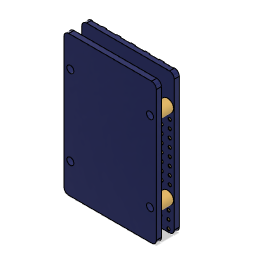
F405wse (Autodesk Fusion 360 design; units mm, degrees)
Autodesk Fusion 360 part; units mm, degrees
note: some values were not read from the file. Set by a fixed rule: which sketch regions a step uses.
sketch "Skizze1" plane through (0, 0, 0) normal (0, 0, 1) x (1, 0, 0)
  line L0 (-14.5, 22) -> (14.5, 22)
  line L1 (14.5, 22) -> (14.5, -22)
  line L2 (14.5, -22) -> (-14.5, -22)
  line L3 (-14.5, -22) -> (-14.5, 22)
  line L4 (-14.5, 22) -> (14.5, -22) construction
  line L5 (14.5, 22) -> (-14.5, -22) construction
  line L6 (-12.5, 12.5) -> (12.5, 12.5) construction
  line L7 (12.5, 12.5) -> (12.5, -12.5) construction
  line L8 (12.5, -12.5) -> (-12.5, -12.5) construction
  line L9 (-12.5, -12.5) -> (-12.5, 12.5) construction
  line L10 (-12.5, 12.5) -> (12.5, -12.5) construction
  line L11 (12.5, 12.5) -> (-12.5, -12.5) construction
  circle A0 centre (-12.5, 12.5) radius 1.1
  circle A1 centre (12.5, 12.5) radius 1.1
  circle A2 centre (12.5, -12.5) radius 1.1
  circle A3 centre (-12.5, -12.5) radius 1.1
  dimension "d1" = 29
  dimension "d2" = 44
  dimension "d7" = 25
  dimension "d8" = 25
  dimension "d9" = 2.2
  constraint horizontal L0
  constraint perpendicular L0 L1
  constraint parallel L0 L2
  constraint parallel L1 L3
  constraint coincident L4 origin
  constraint coincident L5 origin
  constraint horizontal L6
  constraint perpendicular L6 L7
  constraint parallel L6 L8
  constraint parallel L7 L9
  constraint coincident L10 origin
  constraint coincident L11 origin
  constraint coincident L6.start L9.end
  constraint coincident L6.end L7.start
  constraint coincident L7.end L8.start
  constraint coincident L8.end L9.start
  constraint equal A0 A1
  constraint equal A1 A2
  constraint equal A0 A3
  measures "d1" distance of L1.end L2.end
  measures "d2" distance of L0.end L1.end
  measures "d7" distance of L7.end L8.end
  measures "d8" distance of L6.end L7.end
  measures "d9" diameter of A0
extrude "Extrusion1" add sketch "Skizze1" along normal blind 1.2 makes body 1
fillet "Abrundung1" radius 1.5 4 edges at (-14.5, -22, 0.6) (14.5, -22, 0.6) (14.5, 22, 0.6) (-14.5, 22, 0.6) on bodies 1
sketch "Skizze3" plane through (0, 0, 0) normal (0, 0, -1) x (-1, 0, 0)
  arc A0 (14.5, 20.5) -> (13, 22) centre (13, 20.5) ccw
  line L0 (13, 22) -> (-13, 22)
  arc A1 (-13, 22) -> (-14.5, 20.5) centre (-13, 20.5) ccw
  line L1 (-14.5, 20.5) -> (-14.5, -20.5)
  arc A2 (-14.5, -20.5) -> (-13, -22) centre (-13, -20.5) ccw
  line L2 (-13, -22) -> (13, -22)
  arc A3 (13, -22) -> (14.5, -20.5) centre (13, -20.5) ccw
  line L3 (14.5, -20.5) -> (14.5, 20.5)
  circle A4 centre (-12.5, -12.5) radius 1.1
  circle A5 centre (12.5, -12.5) radius 1.1
  circle A6 centre (-12.5, 12.5) radius 1.1
  circle A7 centre (12.5, 12.5) radius 1.1
  line L4 (-0.75, 22) -> (-3.75, 22)
  line L5 (-3.75, 22) -> (-3.75, 19)
  line L6 (-3.75, 19) -> (-0.75, 19)
  line L7 (-0.75, 19) -> (-0.75, 22)
  line L8 (-12.75, 22) -> (-12.75, 19)
  line L9 (-12.75, 19) -> (-9.75, 19)
  line L10 (-9.75, 22) -> (-12.75, 22)
  line L11 (-9.75, 19) -> (-9.75, 22)
  line L12 (-8.25, 22) -> (-8.25, 19)
  line L13 (-8.25, 19) -> (-5.25, 19)
  line L14 (-5.25, 22) -> (-8.25, 22)
  line L15 (-5.25, 19) -> (-5.25, 22)
  line L16 (0.75, 22) -> (0.75, 19)
  line L17 (0.75, 19) -> (3.75, 19)
  line L18 (3.75, 22) -> (0.75, 22)
  line L19 (3.75, 19) -> (3.75, 22)
  line L20 (5.25, 22) -> (5.25, 19)
  line L21 (5.25, 19) -> (8.25, 19)
  line L22 (8.25, 22) -> (5.25, 22)
  line L23 (8.25, 19) -> (8.25, 22)
  line L24 (9.75, 22) -> (9.75, 19)
  line L25 (9.75, 19) -> (12.75, 19)
  line L26 (12.75, 22) -> (9.75, 22)
  line L27 (12.75, 19) -> (12.75, 22)
  circle A8 centre (-8, -1.27) radius 0.5
  circle A9 centre (-8, -8.89) radius 0.5
  circle A10 centre (-10.54, -8.89) radius 0.5
  circle A11 centre (-13.08, -8.89) radius 0.5
  circle A12 centre (-8, -6.35) radius 0.5
  circle A13 centre (-10.54, -6.35) radius 0.5
  circle A14 centre (-13.08, -6.35) radius 0.5
  circle A15 centre (-8, -3.81) radius 0.5
  circle A16 centre (-10.54, -3.81) radius 0.5
  circle A17 centre (-13.08, -3.81) radius 0.5
  circle A18 centre (-10.54, -1.27) radius 0.5
  circle A19 centre (-13.08, -1.27) radius 0.5
  circle A20 centre (-8, 1.27) radius 0.5
  circle A21 centre (-10.54, 1.27) radius 0.5
  circle A22 centre (-13.08, 1.27) radius 0.5
  circle A23 centre (-8, 3.81) radius 0.5
  circle A24 centre (-10.54, 3.81) radius 0.5
  circle A25 centre (-13.08, 3.81) radius 0.5
  circle A26 centre (-8, 6.35) radius 0.5
  circle A27 centre (-10.54, 6.35) radius 0.5
  circle A28 centre (-13.08, 6.35) radius 0.5
  circle A29 centre (-8, 8.89) radius 0.5
  circle A30 centre (-10.54, 8.89) radius 0.5
  circle A31 centre (-13.08, 8.89) radius 0.5
  circle A32 centre (0, -16) radius 0.5
  circle A33 centre (-12.7, -16) radius 0.5
  circle A34 centre (-10.16, -16) radius 0.5
  circle A35 centre (-7.62, -16) radius 0.5
  circle A36 centre (-5.08, -16) radius 0.5
  circle A37 centre (-2.54, -16) radius 0.5
  circle A38 centre (2.54, -16) radius 0.5
  circle A39 centre (5.08, -16) radius 0.5
  circle A40 centre (7.62, -16) radius 0.5
  circle A41 centre (10.16, -16) radius 0.5
  circle A42 centre (12.7, -16) radius 0.5
  circle A43 centre (-12.7, -18.54) radius 0.5
  circle A44 centre (-10.16, -18.54) radius 0.5
  circle A45 centre (-7.62, -18.54) radius 0.5
  circle A46 centre (-5.08, -18.54) radius 0.5
  circle A47 centre (-2.54, -18.54) radius 0.5
  circle A48 centre (0, -18.54) radius 0.5
  circle A49 centre (2.54, -18.54) radius 0.5
  circle A50 centre (5.08, -18.54) radius 0.5
  circle A51 centre (7.62, -18.54) radius 0.5
  circle A52 centre (10.16, -18.54) radius 0.5
  circle A53 centre (12.7, -18.54) radius 0.5
  circle A54 centre (-12.7, -21.08) radius 0.5
  circle A55 centre (-10.16, -21.08) radius 0.5
  circle A56 centre (-7.62, -21.08) radius 0.5
  circle A57 centre (-5.08, -21.08) radius 0.5
  circle A58 centre (-2.54, -21.08) radius 0.5
  circle A59 centre (0, -21.08) radius 0.5
  circle A60 centre (2.54, -21.08) radius 0.5
  circle A61 centre (5.08, -21.08) radius 0.5
  circle A62 centre (7.62, -21.08) radius 0.5
  circle A63 centre (10.16, -21.08) radius 0.5
  circle A64 centre (12.7, -21.08) radius 0.5
  dimension "d33" = 3
  dimension "d34" = 3
  dimension "d35" = 0.75
  dimension "d38" = 4.5
  dimension "d39" = 0
  dimension "d40" = 1
  dimension "d43" = -2.54
  dimension "d44" = 2.54
  dimension "d45" = 1.27
  dimension "d46" = 8
  dimension "d49" = 2.54
  dimension "d50" = -2.54
  dimension "d51" = 16
  constraint horizontal L4
  constraint vertical L5
  constraint horizontal L6
  constraint vertical L7
  constraint coincident L0 L4.start
  constraint equal A8 A32
  constraint vertical origin A32.centre
  measures "d33" distance of L4.start L4.end
  measures "d34" distance of L4.start L6.end
  measures "d35" distance of origin L7
  measures "d40" diameter of A8
  measures "d45" vertical distance of origin A8.centre
  measures "d46" horizontal distance of origin A8.centre
  measures "d51" distance of origin A32.centre
extrude "Extrusion3" add sketch "Skizze3" along normal blind 0.2 contours A0 L0 A1 L1 A2 L2 A3 L3 L5 L6 L7 L8 L9 L11 L12 L13 L15 L16 L17 L19 L20 L21 L23 L24 L25 L27 bodies 1
sketch "Skizze4" plane through (0, 0, 1.2) normal (0, 0, 1) x (1, 0, 0)
  circle A0 centre (-12.5, -12.5) radius 1.1
  circle A1 centre (12.5, -12.5) radius 1.1
  circle A2 centre (12.5, 12.5) radius 1.1
  circle A3 centre (-12.5, 12.5) radius 1.1
  arc A4 (-13, 22) -> (-14.5, 20.5) centre (-13, 20.5) ccw
  line L0 (-14.5, 20.5) -> (-14.5, -20.5)
  arc A5 (-14.5, -20.5) -> (-13, -22) centre (-13, -20.5) ccw
  line L1 (-13, -22) -> (13, -22)
  arc A6 (13, -22) -> (14.5, -20.5) centre (13, -20.5) ccw
  line L2 (14.5, -20.5) -> (14.5, 20.5)
  arc A7 (14.5, 20.5) -> (13, 22) centre (13, 20.5) ccw
  line L3 (13, 22) -> (-13, 22)
  circle A8 centre (12.5, -12.5) radius 1.1
  circle A9 centre (12.5, 12.5) radius 1.1
  circle A10 centre (13.08, -6.35) radius 0.5
  circle A11 centre (10.54, -6.35) radius 0.5
  circle A12 centre (8, -6.35) radius 0.5
  circle A13 centre (8, -1.27) radius 0.5
  circle A14 centre (-12.5, 12.5) radius 1.1
  circle A15 centre (13.08, -8.89) radius 0.5
  circle A16 centre (8, -8.89) radius 0.5
  circle A17 centre (10.54, -8.89) radius 0.5
  circle A18 centre (8, -3.81) radius 0.5
  circle A19 centre (13.08, -3.81) radius 0.5
  circle A20 centre (10.54, -3.81) radius 0.5
  circle A21 centre (-12.5, -12.5) radius 1.1
  circle A22 centre (2.54, -21.08) radius 0.5
  circle A23 centre (12.7, -18.54) radius 0.5
  circle A24 centre (13.08, 8.89) radius 0.5
  circle A25 centre (13.08, 6.35) radius 0.5
  circle A26 centre (5.08, -16) radius 0.5
  circle A27 centre (-5.08, -16) radius 0.5
  circle A28 centre (-7.62, -21.08) radius 0.5
  circle A29 centre (7.62, -21.08) radius 0.5
  circle A30 centre (-12.7, -21.08) radius 0.5
  circle A31 centre (-10.16, -16) radius 0.5
  circle A32 centre (0, -16) radius 0.5
  circle A33 centre (13.08, 3.81) radius 0.5
  circle A34 centre (10.54, 1.27) radius 0.5
  circle A35 centre (13.08, 1.27) radius 0.5
  circle A36 centre (8, 6.35) radius 0.5
  circle A37 centre (7.62, -16) radius 0.5
  circle A38 centre (-5.08, -21.08) radius 0.5
  circle A39 centre (-2.54, -16) radius 0.5
  circle A40 centre (-7.62, -18.54) radius 0.5
  circle A41 centre (10.54, 8.89) radius 0.5
  circle A42 centre (10.54, 6.35) radius 0.5
  circle A43 centre (8, 3.81) radius 0.5
  circle A44 centre (8, 1.27) radius 0.5
  circle A45 centre (10.54, 3.81) radius 0.5
  circle A46 centre (8, 8.89) radius 0.5
  circle A47 centre (2.54, -16) radius 0.5
  circle A48 centre (-2.54, -21.08) radius 0.5
  circle A49 centre (-10.16, -18.54) radius 0.5
  circle A50 centre (12.7, -21.08) radius 0.5
  circle A51 centre (-12.7, -18.54) radius 0.5
  circle A52 centre (10.16, -21.08) radius 0.5
  circle A53 centre (5.08, -21.08) radius 0.5
  circle A54 centre (-10.16, -21.08) radius 0.5
  circle A55 centre (-7.62, -16) radius 0.5
  circle A56 centre (10.16, -16) radius 0.5
  circle A57 centre (10.54, -1.27) radius 0.5
  circle A58 centre (13.08, -1.27) radius 0.5
  circle A59 centre (12.7, -16) radius 0.5
  circle A60 centre (-12.7, -16) radius 0.5
  circle A61 centre (0, -21.08) radius 0.5
  circle A62 centre (-5.08, -18.54) radius 0.5
  circle A63 centre (7.62, -18.54) radius 0.5
  circle A64 centre (5.08, -18.54) radius 0.5
  circle A65 centre (-2.54, -18.54) radius 0.5
  circle A66 centre (2.54, -18.54) radius 0.5
  circle A67 centre (0, -18.54) radius 0.5
  circle A68 centre (10.16, -18.54) radius 0.5
  line L4 (-9.75, 22) -> (-8.25, 22)
  line L5 (-8.25, 22) -> (-8.25, 19)
  line L6 (-8.25, 19) -> (-5.25, 19)
  line L7 (-5.25, 19) -> (-5.25, 22)
  line L8 (-5.25, 22) -> (-3.75, 22)
  line L9 (-3.75, 22) -> (-3.75, 19)
  line L10 (-3.75, 19) -> (-0.75, 19)
  line L11 (-0.75, 19) -> (-0.75, 22)
  line L12 (-0.75, 22) -> (0.75, 22)
  line L13 (0.75, 22) -> (0.75, 19)
  line L14 (0.75, 19) -> (3.75, 19)
  line L15 (3.75, 19) -> (3.75, 22)
  line L16 (3.75, 22) -> (5.25, 22)
  line L17 (5.25, 22) -> (5.25, 19)
  line L18 (5.25, 19) -> (8.25, 19)
  line L19 (8.25, 19) -> (8.25, 22)
  line L20 (8.25, 22) -> (9.75, 22)
  line L21 (9.75, 22) -> (9.75, 19)
  line L22 (9.75, 19) -> (12.75, 19)
  line L23 (12.75, 19) -> (12.75, 22)
  line L24 (12.75, 22) -> (13, 22)
  arc A69 (14.5, 20.5) -> (13, 22) centre (13, 20.5) ccw
  line L25 (14.5, 20.5) -> (14.5, -20.5)
  arc A70 (13, -22) -> (14.5, -20.5) centre (13, -20.5) ccw
  line L26 (13, -22) -> (-13, -22)
  arc A71 (-14.5, -20.5) -> (-13, -22) centre (-13, -20.5) ccw
  line L27 (-14.5, -20.5) -> (-14.5, 20.5)
  arc A72 (-13, 22) -> (-14.5, 20.5) centre (-13, 20.5) ccw
  line L28 (-13, 22) -> (-12.75, 22)
  line L29 (-12.75, 22) -> (-12.75, 19)
  line L30 (-12.75, 19) -> (-9.75, 19)
  line L31 (-9.75, 19) -> (-9.75, 22)
extrude "Extrusion4" add sketch "Skizze4" along normal blind 0.2 bodies 1
sketch "Skizze5" plane through (0, 0, -0.2) normal (0, 0, -1) x (-1, 0, 0)
  circle A0 centre (-12.5, -12.5) radius 1.1
  circle A1 centre (-12.5, 12.5) radius 1.1
  circle A2 centre (-13.08, -6.35) radius 0.5
  circle A3 centre (-10.54, -6.35) radius 0.5
  circle A4 centre (-8, -6.35) radius 0.5
  circle A5 centre (-8, -1.27) radius 0.5
  circle A6 centre (12.5, 12.5) radius 1.1
  circle A7 centre (-13.08, -8.89) radius 0.5
  circle A8 centre (-8, -8.89) radius 0.5
  circle A9 centre (-10.54, -8.89) radius 0.5
  circle A10 centre (-8, -3.81) radius 0.5
  circle A11 centre (-13.08, -3.81) radius 0.5
  circle A12 centre (-10.54, -3.81) radius 0.5
  circle A13 centre (12.5, -12.5) radius 1.1
  circle A14 centre (-2.54, -21.08) radius 0.5
  circle A15 centre (-12.7, -18.54) radius 0.5
  circle A16 centre (-13.08, 8.89) radius 0.5
  circle A17 centre (-13.08, 6.35) radius 0.5
  circle A18 centre (-5.08, -16) radius 0.5
  circle A19 centre (5.08, -16) radius 0.5
  circle A20 centre (7.62, -21.08) radius 0.5
  circle A21 centre (-7.62, -21.08) radius 0.5
  circle A22 centre (12.7, -21.08) radius 0.5
  circle A23 centre (10.16, -16) radius 0.5
  circle A24 centre (0, -16) radius 0.5
  circle A25 centre (-13.08, 3.81) radius 0.5
  circle A26 centre (-10.54, 1.27) radius 0.5
  circle A27 centre (-13.08, 1.27) radius 0.5
  circle A28 centre (-8, 6.35) radius 0.5
  circle A29 centre (-7.62, -16) radius 0.5
  circle A30 centre (5.08, -21.08) radius 0.5
  circle A31 centre (2.54, -16) radius 0.5
  circle A32 centre (7.62, -18.54) radius 0.5
  circle A33 centre (-10.54, 8.89) radius 0.5
  circle A34 centre (-10.54, 6.35) radius 0.5
  circle A35 centre (-8, 3.81) radius 0.5
  circle A36 centre (-8, 1.27) radius 0.5
  circle A37 centre (-10.54, 3.81) radius 0.5
  circle A38 centre (-8, 8.89) radius 0.5
  circle A39 centre (-2.54, -16) radius 0.5
  circle A40 centre (2.54, -21.08) radius 0.5
  circle A41 centre (10.16, -18.54) radius 0.5
  circle A42 centre (-12.7, -21.08) radius 0.5
  circle A43 centre (12.7, -18.54) radius 0.5
  circle A44 centre (-10.16, -21.08) radius 0.5
  circle A45 centre (-5.08, -21.08) radius 0.5
  circle A46 centre (10.16, -21.08) radius 0.5
  circle A47 centre (7.62, -16) radius 0.5
  circle A48 centre (-10.16, -16) radius 0.5
  circle A49 centre (-10.54, -1.27) radius 0.5
  circle A50 centre (-13.08, -1.27) radius 0.5
  circle A51 centre (-12.7, -16) radius 0.5
  circle A52 centre (12.7, -16) radius 0.5
  circle A53 centre (0, -21.08) radius 0.5
  circle A54 centre (5.08, -18.54) radius 0.5
  circle A55 centre (-7.62, -18.54) radius 0.5
  circle A56 centre (-5.08, -18.54) radius 0.5
  circle A57 centre (2.54, -18.54) radius 0.5
  circle A58 centre (-2.54, -18.54) radius 0.5
  circle A59 centre (0, -18.54) radius 0.5
  circle A60 centre (-10.16, -18.54) radius 0.5
  line L0 (9.75, 22) -> (8.25, 22)
  line L1 (8.25, 22) -> (8.25, 19)
  line L2 (8.25, 19) -> (5.25, 19)
  line L3 (5.25, 19) -> (5.25, 22)
  line L4 (5.25, 22) -> (3.75, 22)
  line L5 (3.75, 22) -> (3.75, 19)
  line L6 (3.75, 19) -> (0.75, 19)
  line L7 (0.75, 19) -> (0.75, 22)
  line L8 (0.75, 22) -> (-0.75, 22)
  line L9 (-0.75, 22) -> (-0.75, 19)
  line L10 (-0.75, 19) -> (-3.75, 19)
  line L11 (-3.75, 19) -> (-3.75, 22)
  line L12 (-3.75, 22) -> (-5.25, 22)
  line L13 (-5.25, 22) -> (-5.25, 19)
  line L14 (-5.25, 19) -> (-8.25, 19)
  line L15 (-8.25, 19) -> (-8.25, 22)
  line L16 (-8.25, 22) -> (-9.75, 22)
  line L17 (-9.75, 22) -> (-9.75, 19)
  line L18 (-9.75, 19) -> (-12.75, 19)
  line L19 (-12.75, 19) -> (-12.75, 22)
  line L20 (-12.75, 22) -> (-13, 22)
  arc A61 (-13, 22) -> (-14.5, 20.5) centre (-13, 20.5) ccw
  line L21 (-14.5, 20.5) -> (-14.5, -20.5)
  arc A62 (-14.5, -20.5) -> (-13, -22) centre (-13, -20.5) ccw
  line L22 (-13, -22) -> (13, -22)
  arc A63 (13, -22) -> (14.5, -20.5) centre (13, -20.5) ccw
  line L23 (14.5, -20.5) -> (14.5, 20.5)
  arc A64 (14.5, 20.5) -> (13, 22) centre (13, 20.5) ccw
  line L24 (13, 22) -> (12.75, 22)
  line L25 (12.75, 22) -> (12.75, 19)
  line L26 (12.75, 19) -> (9.75, 19)
  line L27 (9.75, 19) -> (9.75, 22)
  line L28 (1, 6) -> (13, 6)
  line L29 (13, 6) -> (13, -6)
  line L30 (13, -6) -> (1, -6)
  line L31 (1, -6) -> (1, 6)
  dimension "d56" = 12
  dimension "d57" = 6
  dimension "d58" = 1
  constraint horizontal L28
  constraint vertical L29
  constraint horizontal L30
  constraint vertical L31
  constraint equal L28 L31
  measures "d56" distance of L28.start L28.end
  measures "d57" distance of origin L28
  measures "d58" distance of origin L31
extrude "Extrusion5" add sketch "Skizze5" along normal blind 2 contours L28 L29 L30 L31 bodies 1
chamfer "Fase1" distance 0.5 angle 45 4 edges at (-7, -6, -0.2) (-1, 0, -0.2) (-13, 0, -0.2) (-7, 6, -0.2) on bodies 1
sketch "Skizze6" plane through (0, 0, -0.2) normal (0, 0, -1) x (-1, 0, 0)
  line L0 (9.75, 22) -> (8.25, 22)
  line L1 (8.25, 22) -> (8.25, 19)
  line L2 (8.25, 19) -> (5.25, 19)
  line L3 (5.25, 19) -> (5.25, 22)
  line L4 (5.25, 22) -> (3.75, 22)
  line L5 (3.75, 22) -> (3.75, 19)
  line L6 (3.75, 19) -> (0.75, 19)
  line L7 (0.75, 19) -> (0.75, 22)
  line L8 (0.75, 22) -> (-0.75, 22)
  line L9 (-0.75, 22) -> (-0.75, 19)
  line L10 (-0.75, 19) -> (-3.75, 19)
  line L11 (-3.75, 19) -> (-3.75, 22)
  line L12 (-3.75, 22) -> (-5.25, 22)
  line L13 (-5.25, 22) -> (-5.25, 19)
  line L14 (-5.25, 19) -> (-8.25, 19)
  line L15 (-8.25, 19) -> (-8.25, 22)
  line L16 (-8.25, 22) -> (-9.75, 22)
  line L17 (-9.75, 22) -> (-9.75, 19)
  line L18 (-9.75, 19) -> (-12.75, 19)
  line L19 (-12.75, 19) -> (-12.75, 22)
  line L20 (-12.75, 22) -> (-13, 22)
  arc A0 (-13, 22) -> (-14.5, 20.5) centre (-13, 20.5) ccw
  line L21 (-14.5, 20.5) -> (-14.5, -20.5)
  arc A1 (-14.5, -20.5) -> (-13, -22) centre (-13, -20.5) ccw
  line L22 (-13, -22) -> (13, -22)
  arc A2 (13, -22) -> (14.5, -20.5) centre (13, -20.5) ccw
  line L23 (14.5, -20.5) -> (14.5, 20.5)
  arc A3 (14.5, 20.5) -> (13, 22) centre (13, 20.5) ccw
  line L24 (13, 22) -> (12.75, 22)
  line L25 (12.75, 22) -> (12.75, 19)
  line L26 (12.75, 19) -> (9.75, 19)
  line L27 (9.75, 19) -> (9.75, 22)
  circle A4 centre (-10.16, -18.54) radius 0.5
  circle A5 centre (0, -18.54) radius 0.5
  circle A6 centre (-2.54, -18.54) radius 0.5
  circle A7 centre (2.54, -18.54) radius 0.5
  circle A8 centre (-5.08, -18.54) radius 0.5
  circle A9 centre (-7.62, -18.54) radius 0.5
  circle A10 centre (5.08, -18.54) radius 0.5
  circle A11 centre (0, -21.08) radius 0.5
  circle A12 centre (12.7, -16) radius 0.5
  circle A13 centre (-12.7, -16) radius 0.5
  circle A14 centre (-13.08, -1.27) radius 0.5
  circle A15 centre (-10.54, -1.27) radius 0.5
  circle A16 centre (-10.16, -16) radius 0.5
  circle A17 centre (7.62, -16) radius 0.5
  circle A18 centre (10.16, -21.08) radius 0.5
  circle A19 centre (-5.08, -21.08) radius 0.5
  circle A20 centre (-10.16, -21.08) radius 0.5
  circle A21 centre (12.7, -18.54) radius 0.5
  circle A22 centre (-12.7, -21.08) radius 0.5
  circle A23 centre (10.16, -18.54) radius 0.5
  circle A24 centre (2.54, -21.08) radius 0.5
  circle A25 centre (-2.54, -16) radius 0.5
  circle A26 centre (-8, 8.89) radius 0.5
  circle A27 centre (-10.54, 3.81) radius 0.5
  circle A28 centre (-8, 1.27) radius 0.5
  circle A29 centre (-8, 3.81) radius 0.5
  circle A30 centre (-10.54, 6.35) radius 0.5
  circle A31 centre (-10.54, 8.89) radius 0.5
  circle A32 centre (7.62, -18.54) radius 0.5
  circle A33 centre (2.54, -16) radius 0.5
  circle A34 centre (5.08, -21.08) radius 0.5
  circle A35 centre (-7.62, -16) radius 0.5
  circle A36 centre (-8, 6.35) radius 0.5
  circle A37 centre (-13.08, 1.27) radius 0.5
  circle A38 centre (-10.54, 1.27) radius 0.5
  circle A39 centre (-13.08, 3.81) radius 0.5
  circle A40 centre (0, -16) radius 0.5
  circle A41 centre (10.16, -16) radius 0.5
  circle A42 centre (12.7, -21.08) radius 0.5
  circle A43 centre (-7.62, -21.08) radius 0.5
  circle A44 centre (7.62, -21.08) radius 0.5
  circle A45 centre (5.08, -16) radius 0.5
  circle A46 centre (-5.08, -16) radius 0.5
  circle A47 centre (-13.08, 6.35) radius 0.5
  circle A48 centre (-13.08, 8.89) radius 0.5
  circle A49 centre (-12.7, -18.54) radius 0.5
  circle A50 centre (-2.54, -21.08) radius 0.5
  circle A51 centre (12.5, -12.5) radius 1.1
  circle A52 centre (-10.54, -3.81) radius 0.5
  circle A53 centre (-13.08, -3.81) radius 0.5
  circle A54 centre (-8, -3.81) radius 0.5
  circle A55 centre (-10.54, -8.89) radius 0.5
  circle A56 centre (-8, -8.89) radius 0.5
  circle A57 centre (-13.08, -8.89) radius 0.5
  circle A58 centre (12.5, 12.5) radius 1.1
  circle A59 centre (-8, -1.27) radius 0.5
  circle A60 centre (-8, -6.35) radius 0.5
  circle A61 centre (-10.54, -6.35) radius 0.5
  circle A62 centre (-13.08, -6.35) radius 0.5
  circle A63 centre (-12.5, 12.5) radius 1.1
  circle A64 centre (-12.5, -12.5) radius 1.1
  line L28 (13.5, 6.5) -> (13.5, -6.5)
  line L29 (13.5, -6.5) -> (0.5, -6.5)
  line L30 (0.5, -6.5) -> (0.5, 6.5)
  line L31 (0.5, 6.5) -> (13.5, 6.5)
  line L32 (-6, 4) -> (-1, 4)
  line L33 (-1, 4) -> (-1, -8)
  line L34 (-1, -8) -> (-6, -8)
  line L35 (-6, -8) -> (-6, 4)
  dimension "d62" = 12
  dimension "d63" = 5
  dimension "d64" = 1
  dimension "d65" = 4
  constraint horizontal L32
  constraint vertical L33
  constraint horizontal L34
  constraint vertical L35
  measures "d62" distance of L32.start L34.end
  measures "d63" distance of L32.start L32.end
  measures "d64" distance of origin L33
  measures "d65" distance of origin L32
extrude "Extrusion6" add sketch "Skizze6" along normal blind 4 contours L32 L33 L34 L35 bodies 1
sketch "Skizze7" plane through (0, 0, 1.4) normal (0, 0, 1) x (1, 0, 0)
  circle A0 centre (-7.62, -21.08) radius 0.5
  circle A1 centre (12.5, -12.5) radius 1.1
  circle A2 centre (8, 8.89) radius 0.5
  circle A3 centre (8, 6.35) radius 0.5
  circle A4 centre (-10.16, -18.54) radius 0.5
  circle A5 centre (12.7, -21.08) radius 0.5
  circle A6 centre (10.16, -21.08) radius 0.5
  circle A7 centre (10.54, 3.81) radius 0.5
  circle A8 centre (7.62, -18.54) radius 0.5
  circle A9 centre (-12.5, 12.5) radius 1.1
  circle A10 centre (10.54, 1.27) radius 0.5
  circle A11 centre (-2.54, -16) radius 0.5
  circle A12 centre (10.54, 8.89) radius 0.5
  circle A13 centre (8, 3.81) radius 0.5
  circle A14 centre (5.08, -16) radius 0.5
  circle A15 centre (13.08, -6.35) radius 0.5
  circle A16 centre (12.7, -18.54) radius 0.5
  circle A17 centre (12.7, -16) radius 0.5
  circle A18 centre (-10.16, -16) radius 0.5
  circle A19 centre (0, -21.08) radius 0.5
  circle A20 centre (-12.7, -18.54) radius 0.5
  circle A21 centre (-2.54, -21.08) radius 0.5
  circle A22 centre (2.54, -16) radius 0.5
  circle A23 centre (8, -6.35) radius 0.5
  circle A24 centre (2.54, -21.08) radius 0.5
  circle A25 centre (-12.7, -21.08) radius 0.5
  circle A26 centre (13.08, 8.89) radius 0.5
  circle A27 centre (10.54, -6.35) radius 0.5
  circle A28 centre (8, -1.27) radius 0.5
  circle A29 centre (5.08, -18.54) radius 0.5
  circle A30 centre (8, -3.81) radius 0.5
  circle A31 centre (8, -8.89) radius 0.5
  circle A32 centre (13.08, 1.27) radius 0.5
  circle A33 centre (13.08, -8.89) radius 0.5
  circle A34 centre (0, -16) radius 0.5
  circle A35 centre (-5.08, -16) radius 0.5
  circle A36 centre (13.08, -3.81) radius 0.5
  circle A37 centre (-12.7, -16) radius 0.5
  circle A38 centre (7.62, -16) radius 0.5
  circle A39 centre (7.62, -21.08) radius 0.5
  circle A40 centre (-12.5, -12.5) radius 1.1
  circle A41 centre (13.08, -1.27) radius 0.5
  circle A42 centre (-5.08, -18.54) radius 0.5
  circle A43 centre (10.54, -3.81) radius 0.5
  circle A44 centre (10.16, -18.54) radius 0.5
  circle A45 centre (10.54, -8.89) radius 0.5
  circle A46 centre (13.08, 6.35) radius 0.5
  circle A47 centre (13.08, 3.81) radius 0.5
  circle A48 centre (-5.08, -21.08) radius 0.5
  circle A49 centre (-7.62, -18.54) radius 0.5
  circle A50 centre (10.54, 6.35) radius 0.5
  circle A51 centre (8, 1.27) radius 0.5
  circle A52 centre (-2.54, -18.54) radius 0.5
  circle A53 centre (10.54, -1.27) radius 0.5
  circle A54 centre (5.08, -21.08) radius 0.5
  circle A55 centre (2.54, -18.54) radius 0.5
  circle A56 centre (-10.16, -21.08) radius 0.5
  circle A57 centre (10.16, -16) radius 0.5
  circle A58 centre (-7.62, -16) radius 0.5
  circle A59 centre (0, -18.54) radius 0.5
  circle A60 centre (12.5, 12.5) radius 1.1
  arc A61 (-14.5, -20.5) -> (-13, -22) centre (-13, -20.5) ccw
  line L0 (-13, -22) -> (13, -22)
  arc A62 (13, -22) -> (14.5, -20.5) centre (13, -20.5) ccw
  line L1 (14.5, -20.5) -> (14.5, 20.5)
  arc A63 (14.5, 20.5) -> (13, 22) centre (13, 20.5) ccw
  line L2 (13, 22) -> (-13, 22)
  arc A64 (-13, 22) -> (-14.5, 20.5) centre (-13, 20.5) ccw
  line L3 (-14.5, 20.5) -> (-14.5, -20.5)
  line L4 (-14.5, 10.5) -> (-11.5, 10.5)
  line L5 (-11.5, 10.5) -> (-11.5, 2.5)
  line L6 (-11.5, 2.5) -> (-14.5, 2.5)
  line L7 (-14.5, 2.5) -> (-14.5, 10.5)
  line L8 (-14.5, -2.5) -> (-11.5, -2.5)
  line L9 (-11.5, -2.5) -> (-11.5, -10.5)
  line L10 (-11.5, -10.5) -> (-14.5, -10.5)
  line L11 (-14.5, -10.5) -> (-14.5, -2.5)
  line L12 (0, 0) -> (-14.5, 0) construction
  line L13 (-14.4, 10.5) -> (-14.4, 2.5)
  line L14 (-14.4, 2.5) -> (-14.4, -10.5)
  dimension "d68" = 8
  dimension "d69" = 3
  dimension "d70" = 2.5
  dimension "d79" = 0.1
  constraint horizontal L4
  constraint vertical L5
  constraint horizontal L6
  constraint vertical L7
  constraint coincident L3 L4.start
  constraint horizontal L8
  constraint vertical L9
  constraint horizontal L10
  constraint vertical L11
  constraint coincident L3 L8.start
  constraint collinear L5 L9
  constraint coincident L12.start origin
  constraint midpoint L3 L12.end
  constraint symmetric L5 L9 L12
  constraint symmetric L6 L8 L12
  constraint equal L5 L9
  constraint coincident L4 L13.start
  constraint coincident L6 L13.end
  constraint perpendicular L6 L13
  constraint coincident L10 L14.end
  constraint perpendicular L10 L14
  measures "d68" distance of L4.end L5.end
  measures "d69" distance of L5.end L6.end
  measures "d70" distance of L6 L12
  measures "d79" distance of L7 L13
extrude "Extrusion7" add sketch "Skizze7" along normal blind 3 contours L8 L9 L10 L14 | L4 L5 L6 L13 bodies 1
sketch "Skizze8" plane through (0, 0, 1.4) normal (0, 0, 1) x (1, 0, 0)
  circle A0 centre (-7.62, -21.08) radius 0.5
  circle A1 centre (12.5, -12.5) radius 1.1
  circle A2 centre (8, 8.89) radius 0.5
  circle A3 centre (8, 6.35) radius 0.5
  circle A4 centre (-10.16, -18.54) radius 0.5
  circle A5 centre (12.7, -21.08) radius 0.5
  circle A6 centre (10.16, -21.08) radius 0.5
  circle A7 centre (10.54, 3.81) radius 0.5
  circle A8 centre (7.62, -18.54) radius 0.5
  circle A9 centre (-12.5, 12.5) radius 1.1
  circle A10 centre (10.54, 1.27) radius 0.5
  circle A11 centre (-2.54, -16) radius 0.5
  circle A12 centre (10.54, 8.89) radius 0.5
  circle A13 centre (8, 3.81) radius 0.5
  circle A14 centre (5.08, -16) radius 0.5
  circle A15 centre (13.08, -6.35) radius 0.5
  circle A16 centre (12.7, -18.54) radius 0.5
  circle A17 centre (12.7, -16) radius 0.5
  circle A18 centre (-10.16, -16) radius 0.5
  circle A19 centre (0, -21.08) radius 0.5
  circle A20 centre (-12.7, -18.54) radius 0.5
  circle A21 centre (-2.54, -21.08) radius 0.5
  circle A22 centre (2.54, -16) radius 0.5
  circle A23 centre (8, -6.35) radius 0.5
  circle A24 centre (2.54, -21.08) radius 0.5
  circle A25 centre (-12.7, -21.08) radius 0.5
  circle A26 centre (13.08, 8.89) radius 0.5
  circle A27 centre (10.54, -6.35) radius 0.5
  circle A28 centre (8, -1.27) radius 0.5
  circle A29 centre (5.08, -18.54) radius 0.5
  circle A30 centre (8, -3.81) radius 0.5
  circle A31 centre (8, -8.89) radius 0.5
  circle A32 centre (13.08, 1.27) radius 0.5
  circle A33 centre (13.08, -8.89) radius 0.5
  circle A34 centre (0, -16) radius 0.5
  circle A35 centre (-5.08, -16) radius 0.5
  circle A36 centre (13.08, -3.81) radius 0.5
  circle A37 centre (-12.7, -16) radius 0.5
  circle A38 centre (7.62, -16) radius 0.5
  circle A39 centre (7.62, -21.08) radius 0.5
  circle A40 centre (-12.5, -12.5) radius 1.1
  circle A41 centre (13.08, -1.27) radius 0.5
  circle A42 centre (-5.08, -18.54) radius 0.5
  circle A43 centre (10.54, -3.81) radius 0.5
  circle A44 centre (10.16, -18.54) radius 0.5
  circle A45 centre (10.54, -8.89) radius 0.5
  circle A46 centre (13.08, 6.35) radius 0.5
  circle A47 centre (13.08, 3.81) radius 0.5
  circle A48 centre (-5.08, -21.08) radius 0.5
  circle A49 centre (-7.62, -18.54) radius 0.5
  circle A50 centre (10.54, 6.35) radius 0.5
  circle A51 centre (8, 1.27) radius 0.5
  circle A52 centre (-2.54, -18.54) radius 0.5
  circle A53 centre (10.54, -1.27) radius 0.5
  circle A54 centre (5.08, -21.08) radius 0.5
  circle A55 centre (2.54, -18.54) radius 0.5
  circle A56 centre (-10.16, -21.08) radius 0.5
  circle A57 centre (10.16, -16) radius 0.5
  circle A58 centre (-7.62, -16) radius 0.5
  circle A59 centre (0, -18.54) radius 0.5
  circle A60 centre (12.5, 12.5) radius 1.1
  line L0 (-14.4, -2.5) -> (-11.5, -2.5)
  line L1 (-11.5, -2.5) -> (-11.5, -10.5)
  line L2 (-11.5, -10.5) -> (-14.4, -10.5)
  arc A61 (-14.5, -20.5) -> (-13, -22) centre (-13, -20.5) ccw
  line L3 (-13, -22) -> (13, -22)
  arc A62 (13, -22) -> (14.5, -20.5) centre (13, -20.5) ccw
  line L4 (14.5, -20.5) -> (14.5, 20.5)
  arc A63 (14.5, 20.5) -> (13, 22) centre (13, 20.5) ccw
  line L5 (13, 22) -> (-13, 22)
  arc A64 (-13, 22) -> (-14.5, 20.5) centre (-13, 20.5) ccw
  line L6 (-14.5, 20.5) -> (-14.5, -20.5)
  line L7 (-14.4, 10.5) -> (-11.5, 10.5)
  line L8 (-11.5, 10.5) -> (-11.5, 2.5)
  line L9 (-11.5, 2.5) -> (-14.4, 2.5)
  line L10 (-10, 2.5) -> (0, 2.5)
  line L11 (0, 2.5) -> (0, 12.5)
  line L12 (0, 12.5) -> (-10, 12.5)
  line L13 (-10, 12.5) -> (-10, 2.5)
  line L14 (-14.4, -10.5) -> (-14.4, -2.5)
  line L15 (-14.4, 2.5) -> (-14.4, 10.5)
  dimension "d73" = 10
  constraint horizontal L10
  constraint vertical L11
  constraint horizontal L12
  constraint vertical L13
  constraint equal L12 L13
  constraint coincident origin L11
  constraint coincident L8.end L10
  measures "d73" distance of L11.end L12.end
extrude "Extrusion8" add sketch "Skizze8" along normal blind 3.5 contours L10 L11 L12 L13 bodies 1
ref_plane "Arbeitsebene1" through (0, 0, 5.4) normal (0, 0, 1) x (1, 0, 0)
sketch "Skizze9" plane through (0, 0, 5.4) normal (0, 0, 1) x (1, 0, 0)
  line L0 (-10, 12.5) -> (0, 12.5)
  line L1 (0, 12.5) -> (0, 2.5)
  line L2 (0, 2.5) -> (-10, 2.5)
  line L3 (-10, 2.5) -> (-10, 12.5)
  circle A0 centre (-7.62, -21.08) radius 0.5
  circle A1 centre (12.5, -12.5) radius 1.1
  circle A2 centre (8, 8.89) radius 0.5
  circle A3 centre (8, 6.35) radius 0.5
  circle A4 centre (-10.16, -18.54) radius 0.5
  circle A5 centre (12.7, -21.08) radius 0.5
  circle A6 centre (10.16, -21.08) radius 0.5
  circle A7 centre (10.54, 3.81) radius 0.5
  circle A8 centre (7.62, -18.54) radius 0.5
  circle A9 centre (-12.5, 12.5) radius 1.1
  circle A10 centre (10.54, 1.27) radius 0.5
  circle A11 centre (-2.54, -16) radius 0.5
  circle A12 centre (10.54, 8.89) radius 0.5
  circle A13 centre (8, 3.81) radius 0.5
  circle A14 centre (5.08, -16) radius 0.5
  circle A15 centre (13.08, -6.35) radius 0.5
  circle A16 centre (12.7, -18.54) radius 0.5
  circle A17 centre (12.7, -16) radius 0.5
  circle A18 centre (-10.16, -16) radius 0.5
  circle A19 centre (0, -21.08) radius 0.5
  circle A20 centre (-12.7, -18.54) radius 0.5
  circle A21 centre (-2.54, -21.08) radius 0.5
  circle A22 centre (2.54, -16) radius 0.5
  circle A23 centre (8, -6.35) radius 0.5
  circle A24 centre (2.54, -21.08) radius 0.5
  circle A25 centre (-12.7, -21.08) radius 0.5
  circle A26 centre (13.08, 8.89) radius 0.5
  circle A27 centre (10.54, -6.35) radius 0.5
  circle A28 centre (8, -1.27) radius 0.5
  circle A29 centre (5.08, -18.54) radius 0.5
  circle A30 centre (8, -3.81) radius 0.5
  circle A31 centre (8, -8.89) radius 0.5
  circle A32 centre (13.08, 1.27) radius 0.5
  circle A33 centre (13.08, -8.89) radius 0.5
  circle A34 centre (0, -16) radius 0.5
  circle A35 centre (-5.08, -16) radius 0.5
  circle A36 centre (13.08, -3.81) radius 0.5
  circle A37 centre (-12.7, -16) radius 0.5
  circle A38 centre (7.62, -16) radius 0.5
  circle A39 centre (7.62, -21.08) radius 0.5
  circle A40 centre (-12.5, -12.5) radius 1.1
  circle A41 centre (13.08, -1.27) radius 0.5
  circle A42 centre (-5.08, -18.54) radius 0.5
  circle A43 centre (10.54, -3.81) radius 0.5
  circle A44 centre (10.16, -18.54) radius 0.5
  circle A45 centre (10.54, -8.89) radius 0.5
  circle A46 centre (13.08, 6.35) radius 0.5
  circle A47 centre (13.08, 3.81) radius 0.5
  circle A48 centre (-5.08, -21.08) radius 0.5
  circle A49 centre (-7.62, -18.54) radius 0.5
  circle A50 centre (10.54, 6.35) radius 0.5
  circle A51 centre (8, 1.27) radius 0.5
  circle A52 centre (-2.54, -18.54) radius 0.5
  circle A53 centre (10.54, -1.27) radius 0.5
  circle A54 centre (5.08, -21.08) radius 0.5
  circle A55 centre (2.54, -18.54) radius 0.5
  circle A56 centre (-10.16, -21.08) radius 0.5
  circle A57 centre (10.16, -16) radius 0.5
  circle A58 centre (-7.62, -16) radius 0.5
  circle A59 centre (0, -18.54) radius 0.5
  circle A60 centre (12.5, 12.5) radius 1.1
  line L4 (-14.4, -2.5) -> (-11.5, -2.5)
  line L5 (-11.5, -2.5) -> (-11.5, -10.5)
  line L6 (-11.5, -10.5) -> (-14.4, -10.5)
  arc A61 (-14.5, -20.5) -> (-13, -22) centre (-13, -20.5) ccw
  line L7 (-13, -22) -> (13, -22)
  arc A62 (13, -22) -> (14.5, -20.5) centre (13, -20.5) ccw
  line L8 (14.5, -20.5) -> (14.5, 20.5)
  arc A63 (14.5, 20.5) -> (13, 22) centre (13, 20.5) ccw
  line L9 (13, 22) -> (-13, 22)
  arc A64 (-13, 22) -> (-14.5, 20.5) centre (-13, 20.5) ccw
  line L10 (-14.5, 20.5) -> (-14.5, -20.5)
  line L11 (-14.4, 10.5) -> (-11.5, 10.5)
  line L12 (-11.5, 10.5) -> (-11.5, 2.5)
  line L13 (-11.5, 2.5) -> (-14.4, 2.5)
  line L14 (-14.4, 10.5) -> (-14.4, 2.5)
  line L15 (-14.4, -2.5) -> (-14.4, -10.5)
  line L16 (-14.4, -10.5) -> (-14.4, -2.5)
  line L17 (-14.4, 2.5) -> (-14.4, 10.5)
  constraint coincident L11.start L14.start
  constraint coincident L13.end L14.end
  constraint coincident L4.start L15.start
  constraint coincident L6.end L15.end
extrude "Extrusion9" add sketch "Skizze9" along normal blind 1.6 separate body contours L0 L1 L2 L3 | A0 | A2 | A3 | A4 | A5 | A6 | A7 | A8 | A10 | A11 | A12 | A13 | A14 | A15 | A16 | A17 | A18 | A19 | A20 | A21 | A22 | A23 | A24 | A25 | A26 | A27 | A28 | A29 | A30 | A31 | A32 | A33 | A34 | A35 | A36 | A37 | A38 | A39 | A41 | A42 | A43 | A44 | A45 | A46 | A47 | A48 | A49 | A50 | A51 | A52 | A53 | A54 | A55 | A56 | A57 | A58 | A59 | L4 L5 L6 L15 L16 | A61 L7 A62 L8 A63 L9 A64 L10 | L11 L12 L13 L14 L17 makes body 2
sketch "Skizze10" plane through (1, 0, 0) normal (-1, 0, 0) x (0, 0, 1)
  line L0 (-0.2, -8) -> (-0.2, 4)
  line L1 (-0.2, 4) -> (-4.2, 4)
  line L2 (-4.2, 4) -> (-4.2, -8)
  line L3 (-4.2, -8) -> (-0.2, -8)
  line L4 (-3.7, 3.5) -> (-2.7, 3.5)
  line L5 (-2.7, 3.5) -> (-2.7, -7.5)
  line L6 (-2.7, -7.5) -> (-3.7, -7.5)
  line L7 (-3.7, -7.5) -> (-3.7, 3.5)
  dimension "d80" = 0.5
  dimension "d81" = 0.5
  dimension "d82" = 0.5
  dimension "d83" = 1
  constraint horizontal L4
  constraint vertical L5
  constraint horizontal L6
  constraint vertical L7
  measures "d80" distance of L1 L4
  measures "d81" distance of L3 L6
  measures "d82" distance of L2 L7
  measures "d83" distance of L5 L7
extrude "Extrusion10" cut sketch "Skizze10" against normal blind 4.5 contours L4 L5 L6 L7 bodies 1
ref_plane "Arbeitsebene2" through (0, 0, 1.5) normal (0, 0, 1) x (1, 0, 0)
sketch "Skizze11" plane through (0, 0, 1.5) normal (0, 0, 1) x (1, 0, 0)
  circle A0 centre (-12.5, 12.5) radius 1.1
  circle A1 centre (12.5, 12.5) radius 1.1
  circle A2 centre (12.5, -12.5) radius 1.1
  circle A3 centre (-12.5, -12.5) radius 1.1
  circle A4 centre (-12.5, 12.5) radius 1.9
  circle A5 centre (12.5, 12.5) radius 1.9
  circle A6 centre (12.5, -12.5) radius 1.9
  circle A7 centre (-12.5, -12.5) radius 1.9
  dimension "d87" = 3.8
  constraint concentric A0 A4
  constraint concentric A1 A5
  constraint concentric A2 A6
  constraint concentric A3 A7
  constraint equal A6 A7
  constraint equal A5 A6
  constraint equal A4 A5
  measures "d87" diameter of A5
extrude "Extrusion11" add sketch "Skizze11" along normal blind 3.8 separate body makes body 3 at (-10.6024, 12.4053, 4.0333) makes body 4 at (-10.6024, -12.5947, 4.0333) makes body 5 at (14.3976, 12.4053, 4.0333) makes body 6 at (14.3976, -12.5947, 4.0333)
equation "d45 = ( 2.54 / 2 ) * 1 mm"
equation "d57 = d56 / 2"
equation "d81 = d80"
equation "d82 = d80"
